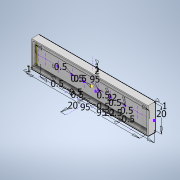
# Autodesk Inventor part: sdm_finger_eit_chamber_mould
Saved by Autodesk Inventor 2021 (Build 250183000, 183)
## iProperties
Created: 2021-05-26
Part Number: sdm_finger_eit_chamber_mould
Material: Generic
Document SubType Name: Modeling
Designer: Charlie
Density: 1 g/cm^3
Appearance: Default
Author: Charlie
Autodesk Inventor part; units mm, degrees
ref_plane "YZ Plane" through (0, 0, 0) normal (1, 0, 0) x (0, 1, 0)
ref_plane "XZ Plane" through (0, 0, 0) normal (0, 1, 0) x (-1, 0, 0)
ref_plane "XY Plane" through (0, 0, 0) normal (0, 0, 1) x (1, 0, 0)
sketch "Sketch2" plane through (0, 0, 0) normal (0, 0, 1) x (1, 0, 0)
  line L0 (-46.5, 10) -> (46.5, 10)
  line L1 (47.5, 9) -> (47.5, -9)
  line L2 (46.5, -10) -> (-46.5, -10)
  line L3 (-47.5, -9) -> (-47.5, 9)
  line L4 (-47.5, 10) -> (47.5, -10) construction
  line L5 (47.5, 10) -> (-47.5, -10) construction
  line L6 (45.5, 8) -> (-45.5, 8)
  line L7 (-45.5, 8) -> (-45.5, -8)
  line L8 (-45.5, -8) -> (45.5, -8)
  line L9 (45.5, -8) -> (45.5, 8)
  line L10 (48.5, 11) -> (-48.5, 11)
  line L11 (-48.5, 11) -> (-48.5, -11)
  line L12 (-48.5, -11) -> (48.5, -11)
  line L13 (48.5, -11) -> (48.5, 11)
  arc A0 (47.5, 9) -> (46.5, 10) centre (46.5, 9) ccw
  arc A1 (46.5, -10) -> (47.5, -9) centre (46.5, -9) ccw
  arc A2 (-47.5, -9) -> (-46.5, -10) centre (-46.5, -9) ccw
  arc A3 (-46.5, 10) -> (-47.5, 9) centre (-46.5, 9) ccw
  point P0 (0, 0)
  dimension "d0" = 95
  dimension "d1" = 20
  dimension "d2" = 2
  dimension "d3" = 1
  dimension "d10" = 1
  constraints: 28 end point, 8 point on circle, 8 point on line, 8 tangent, 6 parallel, 4 centre point, 3 equal radius, 3 perpendicular, 2 midpoint, 1 horizontal, 6 other
  measures "d0" distance of L4.end L5.end
  measures "d1" distance of L5.start L4.end
  measures "d2" distance between parallel lines of L0 L6
  measures "d3" distance between parallel lines of L0 L10
  measures "d10" radius of A0
extrude "Extrusion1" add sketch "Sketch2" along normal blind 1 contours L0 A0 L1 A1 L2 A2 L3 A3 | L9 L8 L7 L6 | L13 L12 L11 L10
extrude "Extrusion2" add sketch "Sketch2" along normal blind 6 contours L13 L12 L11 L10
extrude "Extrusion3" add sketch "Sketch2" along normal blind 4 contours L9 L8 L7 L6
sketch "Sketch3" plane through (-48.5, -11, 0) normal (0, -1, 0) x (1, 0, 0)
  line L0 (95, 5) -> (0, 5) construction
  line L1 (97, 0) -> (97, 6) projected
  line L2 (0, 6) -> (97, 6)
  line L3 (97, 6) -> (97, 0)
  line L4 (97, 0) -> (0, 0)
  line L5 (0, 0) -> (0, 6)
  line L6 (47.5, 5) -> (47.5, 25) construction
  line L7 (0, 0) -> (0, 6) construction
  line L8 (48.5, 3) -> (48.5, -6.8729) construction
  circle A0 centre (19.1132, 5) radius 0.25
  circle A1 centre (30.8868, 5) radius 0.25
  circle A2 centre (41.1132, 5) radius 0.25
  circle A3 centre (52.8868, 5) radius 0.25
  circle A4 centre (63.1132, 5) radius 0.25
  circle A5 centre (74.8868, 5) radius 0.25
  point P0 (48.5, 0)
  point P1 (85.1132, 5)
  point P2 (8.8868, 5)
  point P3 (0, 5)
  dimension "d15" = 95
  dimension "d16" = 22
  dimension "d18" = 20
  dimension "d19" = 1
  dimension "d20" = 0.5
  dimension "d21" = 0.5
  dimension "d22" = 0.5
  dimension "d23" = 0.5
  dimension "d24" = 0.5
  dimension "d25" = 0.5
  constraints: 14 end point, 6 centre point, 6 coincident, 3 point on line, 2 horizontal, 2 parallel, 2 vertical, 1 midpoint, 1 perpendicular, 6 other
  measures "d15" distance of L0.start L0.end
  measures "d16" distance of point (74.887, 5) point (52.887, 5)
  measures "d18" distance of L6.start L6.end
  measures "d19" distance from line of L2 point (0, 5)
  measures "d20" diameter of A0
  measures "d21" diameter of A1
  measures "d22" diameter of A2
  measures "d23" diameter of A3
  measures "d24" diameter of A4
  measures "d25" diameter of A5
sketch "Sketch4" plane through (0, 0, 4) normal (0, 0, 1) x (1, 0, 0)
  line L0 (47.5, 0) -> (-47.5, 0) construction
  circle A0 centre (-28.3868, 0) radius 0.25
  circle A1 centre (-16.6132, 0) radius 0.25
  circle A2 centre (-6.3868, 0) radius 0.25
  circle A3 centre (5.3868, 0) radius 0.25
  circle A4 centre (15.6132, 0) radius 0.25
  circle A5 centre (27.3868, 0) radius 0.25
  line L1 (-45.5, 8) -> (-45.5, -8) projected
  line L2 (0, 0) -> (0, 21.8037) construction
  point P0 (37.6132, 0)
  point P1 (-38.6132, 0)
  point P2 (51.8861, 1)
  point P3 (3.3861, -2)
  point P4 (-45.1139, 0)
  dimension "d30" = 95
  dimension "d31" = 22
  dimension "d33" = 0.5
  dimension "d34" = 0.5
  dimension "d35" = 0.5
  dimension "d36" = 0.5
  dimension "d37" = 0.5
  dimension "d38" = 0.5
  constraints: 6 centre point, 6 coincident, 4 end point, 2 point on line, 1 horizontal, 1 midpoint, 1 vertical, 6 other
  measures "d30" distance of L0.start L0.end
  measures "d31" distance of point (27.387, 0) point (5.387, 0)
  measures "d33" diameter of A0
  measures "d34" diameter of A1
  measures "d35" diameter of A2
  measures "d36" diameter of A3
  measures "d37" diameter of A4
  measures "d38" diameter of A5
body "Solid1"
